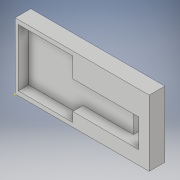
# Autodesk Inventor part: Case
Saved by Autodesk Inventor 2017 (Build 210142000, 142)
## iProperties
Created: 2016-11-30
Part Number: Case
Material: Generic
Document SubType Name: Modeling
Designer: SDL
Density: 1 g/cm^3
Appearance: Default
Author: SDL
Autodesk Inventor part; units mm, degrees
ref_plane "YZ Plane" through (0, 0, 0) normal (1, 0, 0) x (0, 1, 0)
ref_plane "XZ Plane" through (0, 0, 0) normal (0, 1, 0) x (-1, 0, 0)
ref_plane "XY Plane" through (0, 0, 0) normal (0, 0, 1) x (1, 0, 0)
sketch "Sketch3" plane through (0, 0, 0) normal (0, 0, 1) x (1, 0, 0)
  line L0 (3, 4) -> (128, 4)
  line L1 (128, 4) -> (128, 59)
  line L2 (128, 59) -> (3, 59)
  line L3 (3, 59) -> (3, 4)
  point P0 (0, 0)
  dimension "d0" = 125
  dimension "d1" = 55
  constraints: 8 end point, 2 parallel, 1 horizontal, 1 perpendicular
  measures "d0" distance of L2.end L1.end
  measures "d1" distance of L1.end L0.end
extrude "Extrusion1" add sketch "Sketch3" along normal blind 5
sketch "Sketch7" plane through (0, 0, 5) normal (0, 0, 1) x (1, 0, 0)
  line L0 (128, 4) -> (128, 59) projected
  line L1 (0, 4) -> (128, 4) projected
  line L2 (128, 59) -> (53, 59)
  line L3 (53, 59) -> (53, 4)
  line L4 (53, 4) -> (128, 4)
  line L5 (128, 4) -> (128, 59)
  point P0 (0, 0)
  dimension "d20" = 75
  constraints: 8 end point, 2 parallel, 1 horizontal, 1 perpendicular, 2 other
  measures "d20" distance of L4.end L3.end
extrude "Extrusion3" add sketch "Sketch7" along normal blind 10
sketch "Sketch8" plane through (0, 0, 15) normal (0, 0, 1) x (1, 0, 0)
  line L0 (53, 59) -> (53, 4) projected
  line L1 (53, 4) -> (53, 13)
  line L2 (53, 13) -> (118, 13)
  line L3 (118, 13) -> (118, 40)
  line L4 (118, 40) -> (53, 40)
  line L5 (53, 40) -> (53, 13)
  point P0 (0, 0)
  dimension "d23" = 9
  dimension "d24" = 65
  dimension "d25" = 27
  constraints: 10 end point, 2 parallel, 1 horizontal, 1 perpendicular, 1 point on line
  measures "d23" distance of L0.end L1.end
  measures "d24" distance of L4.end L3.end
  measures "d25" distance of L3.end L2.end
extrude "Extrusion4" cut sketch "Sketch8" against normal blind 10
sketch "Sketch9" plane through (0, 0, 15) normal (0, 0, 1) x (1, 0, 0)
  line L0 (53, 40) -> (118, 40) projected
  line L1 (118, 13) -> (53, 13) projected
  line L2 (118, 40) -> (103, 40)
  line L3 (103, 40) -> (103, 13)
  line L4 (103, 13) -> (118, 13)
  line L5 (118, 13) -> (118, 40)
  point P0 (0, 0)
  dimension "d28" = 15
  constraints: 8 end point, 2 parallel, 1 horizontal, 1 perpendicular, 1 point on line
  measures "d28" distance of L4.end L3.end
extrude "Extrusion5" cut sketch "Sketch9" against normal blind 20
sketch "Sketch12" plane through (0, 0, 5) normal (0, 0, 1) x (1, 0, 0)
  line L0 (0, 0) -> (0, 63)
  line L1 (0, 63) -> (128, 63)
  line L2 (128, 63) -> (128, 59)
  line L3 (3, 59) -> (128, 59) projected
  line L4 (128, 59) -> (3, 59)
  line L5 (3, 4) -> (3, 59) projected
  line L6 (3, 59) -> (3, 4)
  line L7 (128, 59) -> (128, 4) projected
  line L8 (3, 4) -> (128, 4)
  line L9 (128, 4) -> (128, 0)
  line L10 (128, 0) -> (0, 0)
  dimension "d35" = 63
  dimension "d36" = 128
  dimension "d37" = 90
  constraints: 16 end point, 4 perpendicular, 2 collinear, 1 point on line, 1 vertical
  measures "d35" distance of L0.start L0.end
  measures "d36" distance of L0.end L1.end
  measures "d37" angle of L0 L1
extrude "Extrusion6" add sketch "Sketch12" along normal blind 10 and the other way blind 5 contours L0 L1 L2 L3 L5 L8 L9 L10
sketch "Sketch14" plane through (0, 0, 5) normal (0, 0, 1) x (1, 0, 0)
  line L0 (53, 40) -> (103, 40) projected
  line L1 (53, 40) -> (55, 40)
  line L2 (55, 40) -> (55, 59)
  line L3 (55, 59) -> (53, 59)
  line L4 (53, 59) -> (53, 40)
  point P0 (0, 0)
  dimension "d42" = 2
  constraints: 8 end point, 2 parallel, 1 horizontal, 1 perpendicular
  measures "d42" distance of L3.end L2.end
extrude "Extrusion7" cut sketch "Sketch14" along normal blind 10
sketch "Sketch15" plane through (0, 0, 15) normal (0, 0, 1) x (1, 0, 0)
  line L0 (53, 4) -> (53, 13) projected
  line L1 (53, 13) -> (55, 13)
  line L2 (55, 13) -> (55, 4)
  line L3 (55, 4) -> (53, 4)
  line L4 (53, 4) -> (53, 13)
  point P0 (0, 0)
  dimension "d45" = 2
  constraints: 8 end point, 2 parallel, 1 horizontal, 1 perpendicular
  measures "d45" distance of L2.end L3.end
extrude "Extrusion8" cut sketch "Sketch15" against normal blind 10
sketch "Sketch17" plane through (0, 0, 15) normal (0, 0, 1) x (1, 0, 0)
  point P0 (0, 0)
body "Solid1"
